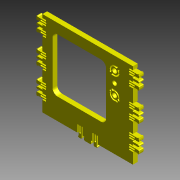
# Autodesk Inventor part: sideA
Saved by Autodesk Inventor 2012 (Build 160160000, 160)
## iProperties
Created: 2011-10-14
Part Number: sideA
Document SubType Name: Modeling
Designer: cramera
Density: 0.952 g/cm^3
Material: High Density Polyethylene
Mass: 352.422 g
Surface Area: 1032.73 cm^2
Volume: 370.191 cm^3
Autodesk Inventor part; units mm, degrees
ref_plane "YZ Plane" through (0, 0, 0) normal (1, 0, 0) x (0, 1, 0)
ref_plane "XZ Plane" through (0, 0, 0) normal (0, 1, 0) x (-1, 0, 0)
ref_plane "XY Plane" through (0, 0, 0) normal (0, 0, 1) x (1, 0, 0)
derived "skeleton.ipt"
sketch "POCKET_1-16" plane through (0, 0, 0) normal (0, 0, 1) x (1, 0, 0)
  circle A0 centre (239.1243, 767.2962) radius 7.3977
  constraints: 1 centre point
sketch "STOCK_12MM" plane through (0, 0, 0) normal (0, 0, 1) x (1, 0, 0)
  line L0 (457.2, 914.4) -> (457.2, 0)
  line L1 (0, 0) -> (457.2, 0)
  line L2 (457.2, 0) -> (457.2, 914.4)
  line L3 (457.2, 914.4) -> (0, 914.4)
  line L4 (0, 914.4) -> (0, 0)
  constraints: 10 end point
sketch "THROUGH-CUT" plane through (0, 0, 0) normal (0, 0, 1) x (1, 0, 0)
  line L0 (94.6618, 802.2212) -> (204.8343, 802.2212)
  arc A0 (217.5343, 789.5212) -> (204.8343, 802.2212) centre (204.8343, 789.5212) ccw
  line L1 (217.5343, 789.5212) -> (217.5343, 678.3962)
  arc A1 (204.8343, 665.6962) -> (217.5343, 678.3962) centre (204.8343, 678.3962) ccw
  line L2 (204.8343, 665.6962) -> (94.6618, 665.6962)
  arc A2 (81.9618, 678.3962) -> (94.6618, 665.6962) centre (94.6618, 678.3962) ccw
  line L3 (81.9618, 678.3962) -> (81.9618, 789.5212)
  arc A3 (94.6618, 802.2212) -> (81.9618, 789.5212) centre (94.6618, 789.5212) ccw
  circle A4 centre (239.1243, 794.2837) radius 5.925
  circle A5 centre (239.1243, 740.3087) radius 5.925
  circle A6 centre (239.1243, 767.2962) radius 5.5563
  arc A7 (51.3833, 713.1307) -> (52.9708, 711.5432) centre (52.9708, 713.1307) ccw
  line L4 (52.9708, 711.5432) -> (64.4993, 711.5432)
  arc A8 (64.4993, 711.5432) -> (66.0868, 713.1307) centre (64.4993, 713.1307) ccw
  line L5 (66.0868, 713.1307) -> (66.0868, 713.2577)
  arc A9 (66.0868, 713.2577) -> (64.4993, 714.8452) centre (64.4993, 713.2577) ccw
  line L6 (64.4993, 714.8452) -> (52.9708, 714.8452)
  arc A10 (52.9708, 714.8452) -> (51.3833, 713.2577) centre (52.9708, 713.2577) ccw
  line L7 (51.3833, 713.2577) -> (51.3833, 713.1307)
  arc A11 (277.2243, 673.8242) -> (275.6368, 672.2367) centre (277.2243, 672.2367) ccw
  line L8 (275.6368, 672.2367) -> (275.6368, 672.1097)
  arc A12 (275.6368, 672.1097) -> (277.2243, 670.5222) centre (277.2243, 672.1097) ccw
  line L9 (277.2243, 670.5222) -> (288.7527, 670.5222)
  arc A13 (288.7527, 670.5222) -> (290.3402, 672.1097) centre (288.7527, 672.1097) ccw
  line L10 (290.3402, 672.1097) -> (290.3402, 672.2367)
  arc A14 (290.3402, 672.2367) -> (288.7527, 673.8242) centre (288.7527, 672.2367) ccw
  line L11 (288.7527, 673.8242) -> (277.2243, 673.8242)
  arc A15 (277.2243, 740.4992) -> (275.6368, 738.9117) centre (277.2243, 738.9117) ccw
  line L12 (275.6368, 738.9117) -> (275.6368, 738.7847)
  arc A16 (275.6368, 738.7847) -> (277.2243, 737.1972) centre (277.2243, 738.7847) ccw
  line L13 (277.2243, 737.1972) -> (288.7527, 737.1972)
  arc A17 (288.7527, 737.1972) -> (290.3402, 738.7847) centre (288.7527, 738.7847) ccw
  line L14 (290.3402, 738.7847) -> (290.3402, 738.9117)
  arc A18 (290.3402, 738.9117) -> (288.7527, 740.4992) centre (288.7527, 738.9117) ccw
  line L15 (288.7527, 740.4992) -> (277.2243, 740.4992)
  line L16 (148.0018, 609.2685) -> (148.0018, 606.6412)
  line L17 (148.0018, 606.6412) -> (146.4778, 605.3712)
  line L18 (146.4778, 605.3712) -> (146.4778, 603.6533)
  line L19 (146.4778, 603.6533) -> (150.0773, 602.8312)
  line L20 (150.0773, 602.8312) -> (153.7803, 602.8312)
  arc A19 (153.7803, 602.8312) -> (155.3678, 604.4187) centre (153.7803, 604.4187) ccw
  line L21 (155.3678, 604.4187) -> (155.3678, 629.1837)
  arc A20 (156.9553, 630.7712) -> (155.3678, 629.1837) centre (156.9553, 629.1837) ccw
  line L22 (156.9553, 630.7712) -> (157.0823, 630.7712)
  arc A21 (158.6698, 629.1837) -> (157.0823, 630.7712) centre (157.0823, 629.1837) ccw
  line L23 (158.6698, 629.1837) -> (158.6698, 611.7212)
  line L24 (158.6698, 611.7212) -> (159.7267, 611.7212)
  arc A22 (161.9718, 609.4762) -> (159.7267, 611.7212) centre (160.8493, 610.5987) ccw
  line L25 (161.9718, 609.4762) -> (161.9718, 604.4187)
  line L26 (161.9718, 604.4187) -> (163.5593, 602.8312)
  line L27 (163.5593, 602.8312) -> (178.1643, 602.8312)
  line L28 (178.1643, 602.8312) -> (179.7518, 604.4187)
  line L29 (179.7518, 604.4187) -> (179.7518, 609.4762)
  arc A23 (181.9968, 611.7212) -> (179.7518, 609.4762) centre (180.8743, 610.5987) ccw
  line L30 (181.9968, 611.7212) -> (183.0538, 611.7212)
  line L31 (183.0538, 611.7212) -> (183.0538, 629.1837)
  arc A24 (184.6413, 630.7712) -> (183.0538, 629.1837) centre (184.6413, 629.1837) ccw
  line L32 (184.6413, 630.7712) -> (184.7604, 630.7712)
  arc A25 (186.3479, 629.1837) -> (184.7604, 630.7712) centre (184.7604, 629.1837) ccw
  line L33 (186.3479, 629.1837) -> (186.3558, 604.4187)
  arc A26 (186.3558, 604.4187) -> (187.9411, 602.8312) centre (187.9433, 604.4187) ccw
  line L34 (187.9411, 602.8312) -> (191.6462, 602.8312)
  line L35 (191.6462, 602.8312) -> (195.2458, 603.6533)
  line L36 (195.2458, 603.6533) -> (195.2458, 605.3712)
  line L37 (195.2458, 605.3712) -> (193.7218, 606.6412)
  line L38 (193.7218, 606.6412) -> (193.7218, 609.2685)
  line L39 (193.7218, 609.2685) -> (193.7218, 629.1837)
  arc A27 (195.3093, 630.7712) -> (193.7218, 629.1837) centre (195.3093, 629.1837) ccw
  line L40 (195.3093, 630.7712) -> (195.4363, 630.7712)
  arc A28 (197.0238, 629.1837) -> (195.4363, 630.7712) centre (195.4363, 629.1837) ccw
  line L41 (197.0238, 629.1837) -> (197.0238, 611.7212)
  line L42 (197.0238, 611.7212) -> (285.5428, 611.7212)
  line L43 (285.5428, 611.7212) -> (285.5428, 639.5342)
  line L44 (285.5428, 639.5342) -> (277.6053, 639.5342)
  arc A29 (276.0178, 641.1217) -> (277.6053, 639.5342) centre (277.6053, 641.1217) ccw
  line L45 (276.0178, 641.1217) -> (276.0178, 641.2487)
  arc A30 (277.6053, 642.8362) -> (276.0178, 641.2487) centre (277.6053, 641.2487) ccw
  line L46 (277.6053, 642.8362) -> (294.3455, 642.8362)
  line L47 (294.3455, 642.8362) -> (296.9728, 642.8362)
  line L48 (296.9728, 642.8362) -> (298.2428, 641.3122)
  line L49 (298.2428, 641.3122) -> (299.9607, 641.3122)
  line L50 (299.9607, 641.3122) -> (300.7828, 644.9118)
  line L51 (300.7828, 644.9118) -> (300.7828, 648.6169)
  arc A31 (300.7828, 648.6169) -> (299.1953, 650.2022) centre (299.1953, 648.6147) ccw
  line L52 (299.1953, 650.2022) -> (277.6053, 650.2022)
  arc A32 (276.0178, 651.7897) -> (277.6053, 650.2022) centre (277.6053, 651.7897) ccw
  line L53 (276.0178, 651.7897) -> (276.0178, 651.9167)
  arc A33 (277.6053, 653.5042) -> (276.0178, 651.9167) centre (277.6053, 651.9167) ccw
  line L54 (277.6053, 653.5042) -> (285.5428, 653.5042)
  line L55 (285.5428, 653.5042) -> (285.5428, 654.5612)
  arc A34 (285.5428, 656.8062) -> (285.5428, 654.5612) centre (286.6653, 655.6837) ccw
  arc A35 (287.7878, 656.8062) -> (285.5428, 656.8062) centre (286.6653, 655.6837) ccw
  line L56 (287.7878, 656.8062) -> (299.1953, 656.8062)
  line L57 (299.1953, 656.8062) -> (300.7828, 658.3937)
  line L58 (300.7828, 658.3937) -> (300.7828, 660.2987)
  line L59 (300.7828, 660.2987) -> (299.1953, 661.8862)
  line L60 (299.1953, 661.8862) -> (287.7878, 661.8862)
  arc A36 (285.5428, 661.8862) -> (287.7878, 661.8862) centre (286.6653, 663.0088) ccw
  arc A37 (285.5428, 664.1313) -> (285.5428, 661.8862) centre (286.6653, 663.0088) ccw
  line L61 (285.5428, 664.1313) -> (285.5428, 665.1882)
  line L62 (285.5428, 665.1882) -> (277.6053, 665.1882)
  arc A38 (276.0178, 666.7757) -> (277.6053, 665.1882) centre (277.6053, 666.7757) ccw
  line L63 (276.0178, 666.7757) -> (276.0178, 666.9027)
  arc A39 (277.6053, 668.4902) -> (276.0178, 666.9027) centre (277.6053, 666.9027) ccw
  line L64 (277.6053, 668.4902) -> (299.1953, 668.4902)
  arc A40 (299.1953, 668.4902) -> (300.7828, 670.0777) centre (299.1953, 670.0777) ccw
  line L65 (300.7828, 670.0777) -> (300.7828, 673.7807)
  line L66 (300.7828, 673.7807) -> (299.9607, 677.3802)
  line L67 (299.9607, 677.3802) -> (298.2428, 677.3802)
  line L68 (298.2428, 677.3802) -> (296.9728, 675.8562)
  line L69 (296.9728, 675.8562) -> (294.3455, 675.8562)
  line L70 (294.3455, 675.8562) -> (277.6053, 675.8562)
  arc A41 (276.0178, 677.4437) -> (277.6053, 675.8562) centre (277.6053, 677.4437) ccw
  line L71 (276.0178, 677.4437) -> (276.0178, 677.5707)
  arc A42 (277.6053, 679.1582) -> (276.0178, 677.5707) centre (277.6053, 677.5707) ccw
  line L72 (277.6053, 679.1582) -> (285.5428, 679.1582)
  line L73 (285.5428, 679.1582) -> (285.5428, 706.2092)
  line L74 (285.5428, 706.2092) -> (277.6053, 706.2092)
  arc A43 (276.0178, 707.7967) -> (277.6053, 706.2092) centre (277.6053, 707.7967) ccw
  line L75 (276.0178, 707.7967) -> (276.0178, 707.9237)
  arc A44 (277.6053, 709.5112) -> (276.0178, 707.9237) centre (277.6053, 707.9237) ccw
  line L76 (277.6053, 709.5112) -> (294.3455, 709.5112)
  line L77 (294.3455, 709.5112) -> (296.9728, 709.5112)
  line L78 (296.9728, 709.5112) -> (298.2428, 707.9872)
  line L79 (298.2428, 707.9872) -> (299.9607, 707.9872)
  line L80 (299.9607, 707.9872) -> (300.7828, 711.5868)
  line L81 (300.7828, 711.5868) -> (300.7828, 715.2919)
  arc A45 (300.7828, 715.2919) -> (299.1953, 716.8772) centre (299.1953, 715.2897) ccw
  line L82 (299.1953, 716.8772) -> (277.6053, 716.8772)
  arc A46 (276.0178, 718.4647) -> (277.6053, 716.8772) centre (277.6053, 718.4647) ccw
  line L83 (276.0178, 718.4647) -> (276.0178, 718.5917)
  arc A47 (277.6053, 720.1792) -> (276.0178, 718.5917) centre (277.6053, 718.5917) ccw
  line L84 (277.6053, 720.1792) -> (285.5428, 720.1792)
  line L85 (285.5428, 720.1792) -> (285.5428, 721.2362)
  arc A48 (285.5428, 723.4812) -> (285.5428, 721.2362) centre (286.6653, 722.3587) ccw
  arc A49 (287.7878, 723.4812) -> (285.5428, 723.4812) centre (286.6653, 722.3587) ccw
  line L86 (287.7878, 723.4812) -> (299.1953, 723.4812)
  line L87 (299.1953, 723.4812) -> (300.7828, 725.0687)
  line L88 (300.7828, 725.0687) -> (300.7828, 726.9737)
  line L89 (300.7828, 726.9737) -> (299.1953, 728.5612)
  line L90 (299.1953, 728.5612) -> (287.7878, 728.5612)
  arc A50 (285.5428, 728.5612) -> (287.7878, 728.5612) centre (286.6653, 729.6838) ccw
  arc A51 (285.5428, 730.8063) -> (285.5428, 728.5612) centre (286.6653, 729.6838) ccw
  line L91 (285.5428, 730.8063) -> (285.5428, 731.8632)
  line L92 (285.5428, 731.8632) -> (277.6053, 731.8632)
  arc A52 (276.0178, 733.4507) -> (277.6053, 731.8632) centre (277.6053, 733.4507) ccw
  line L93 (276.0178, 733.4507) -> (276.0178, 733.5777)
  arc A53 (277.6053, 735.1652) -> (276.0178, 733.5777) centre (277.6053, 733.5777) ccw
  line L94 (277.6053, 735.1652) -> (299.1953, 735.1652)
  arc A54 (299.1953, 735.1652) -> (300.7828, 736.7527) centre (299.1953, 736.7527) ccw
  line L95 (300.7828, 736.7527) -> (300.7828, 740.4557)
  line L96 (300.7828, 740.4557) -> (299.9607, 744.0552)
  line L97 (299.9607, 744.0552) -> (298.2428, 744.0552)
  line L98 (298.2428, 744.0552) -> (296.9728, 742.5312)
  line L99 (296.9728, 742.5312) -> (294.3455, 742.5312)
  line L100 (294.3455, 742.5312) -> (277.6053, 742.5312)
  arc A55 (276.0178, 744.1187) -> (277.6053, 742.5312) centre (277.6053, 744.1187) ccw
  line L101 (276.0178, 744.1187) -> (276.0178, 744.2457)
  arc A56 (277.6053, 745.8332) -> (276.0178, 744.2457) centre (277.6053, 744.2457) ccw
  line L102 (277.6053, 745.8332) -> (285.5428, 745.8332)
  line L103 (285.5428, 745.8332) -> (285.5428, 779.2342)
  line L104 (285.5428, 779.2342) -> (277.6053, 779.2342)
  arc A57 (276.0178, 780.8217) -> (277.6053, 779.2342) centre (277.6053, 780.8217) ccw
  line L105 (276.0178, 780.8217) -> (276.0178, 780.9487)
  arc A58 (277.6053, 782.5362) -> (276.0178, 780.9487) centre (277.6053, 780.9487) ccw
  line L106 (277.6053, 782.5362) -> (294.3455, 782.5362)
  line L107 (294.3455, 782.5362) -> (296.9728, 782.5362)
  line L108 (296.9728, 782.5362) -> (298.2428, 781.0122)
  line L109 (298.2428, 781.0122) -> (299.9607, 781.0122)
  line L110 (299.9607, 781.0122) -> (300.7828, 784.6118)
  line L111 (300.7828, 784.6118) -> (300.7828, 788.3169)
  arc A59 (300.7828, 788.3169) -> (299.1953, 789.9022) centre (299.1953, 788.3147) ccw
  line L112 (299.1953, 789.9022) -> (277.6053, 789.9022)
  arc A60 (276.0178, 791.4897) -> (277.6053, 789.9022) centre (277.6053, 791.4897) ccw
  line L113 (276.0178, 791.4897) -> (276.0178, 791.6167)
  arc A61 (277.6053, 793.2042) -> (276.0178, 791.6167) centre (277.6053, 791.6167) ccw
  line L114 (277.6053, 793.2042) -> (285.5428, 793.2042)
  line L115 (285.5428, 793.2042) -> (285.5428, 794.2612)
  arc A62 (285.5428, 796.5062) -> (285.5428, 794.2612) centre (286.6653, 795.3837) ccw
  arc A63 (287.7878, 796.5062) -> (285.5428, 796.5062) centre (286.6653, 795.3837) ccw
  line L116 (287.7878, 796.5062) -> (299.1953, 796.5062)
  line L117 (299.1953, 796.5062) -> (300.7828, 798.0937)
  line L118 (300.7828, 798.0937) -> (300.7828, 799.9987)
  line L119 (300.7828, 799.9987) -> (299.1953, 801.5862)
  line L120 (299.1953, 801.5862) -> (287.7878, 801.5862)
  arc A64 (285.5428, 801.5862) -> (287.7878, 801.5862) centre (286.6653, 802.7088) ccw
  arc A65 (285.5428, 803.8313) -> (285.5428, 801.5862) centre (286.6653, 802.7088) ccw
  line L121 (285.5428, 803.8313) -> (285.5428, 804.8882)
  line L122 (285.5428, 804.8882) -> (277.6053, 804.8882)
  arc A66 (276.0178, 806.4757) -> (277.6053, 804.8882) centre (277.6053, 806.4757) ccw
  line L123 (276.0178, 806.4757) -> (276.0178, 806.6027)
  arc A67 (277.6053, 808.1902) -> (276.0178, 806.6027) centre (277.6053, 806.6027) ccw
  line L124 (277.6053, 808.1902) -> (299.1953, 808.1902)
  arc A68 (299.1953, 808.1902) -> (300.7828, 809.7777) centre (299.1953, 809.7777) ccw
  line L125 (300.7828, 809.7777) -> (300.7828, 813.4807)
  line L126 (300.7828, 813.4807) -> (299.9607, 817.0802)
  line L127 (299.9607, 817.0802) -> (298.2428, 817.0802)
  line L128 (298.2428, 817.0802) -> (296.9728, 815.5562)
  line L129 (296.9728, 815.5562) -> (294.3455, 815.5562)
  line L130 (294.3455, 815.5562) -> (277.6053, 815.5562)
  arc A69 (276.0178, 817.1437) -> (277.6053, 815.5562) centre (277.6053, 817.1437) ccw
  line L131 (276.0178, 817.1437) -> (276.0178, 817.2707)
  arc A70 (277.6053, 818.8582) -> (276.0178, 817.2707) centre (277.6053, 817.2707) ccw
  line L132 (277.6053, 818.8582) -> (285.5428, 818.8582)
  line L133 (285.5428, 818.8582) -> (285.5428, 827.6212)
  line L134 (285.5428, 827.6212) -> (56.1808, 827.6212)
  line L135 (56.1808, 827.6212) -> (56.1808, 818.8582)
  line L136 (56.1808, 818.8582) -> (65.7058, 818.8582)
  line L137 (65.7058, 818.8582) -> (65.7058, 815.5562)
  line L138 (65.7058, 815.5562) -> (47.3781, 815.5562)
  line L139 (47.3781, 815.5562) -> (44.7508, 815.5562)
  line L140 (44.7508, 815.5562) -> (43.4808, 817.0802)
  line L141 (43.4808, 817.0802) -> (41.7629, 817.0802)
  line L142 (41.7629, 817.0802) -> (40.9408, 813.4807)
  line L143 (40.9408, 813.4807) -> (40.9408, 809.7777)
  arc A71 (40.9408, 809.7777) -> (42.5283, 808.1902) centre (42.5283, 809.7777) ccw
  line L144 (42.5283, 808.1902) -> (64.1183, 808.1902)
  arc A72 (65.7058, 806.6027) -> (64.1183, 808.1902) centre (64.1183, 806.6027) ccw
  line L145 (65.7058, 806.6027) -> (65.7058, 806.4757)
  arc A73 (64.1183, 804.8882) -> (65.7058, 806.4757) centre (64.1183, 806.4757) ccw
  line L146 (64.1183, 804.8882) -> (56.1808, 804.8882)
  line L147 (56.1808, 804.8882) -> (56.1808, 803.8313)
  arc A74 (53.9357, 801.5862) -> (56.1808, 803.8313) centre (55.0583, 802.7088) ccw
  line L148 (53.9357, 801.5862) -> (42.5283, 801.5862)
  line L149 (42.5283, 801.5862) -> (40.9408, 799.9987)
  line L150 (40.9408, 799.9987) -> (40.9408, 798.0937)
  line L151 (40.9408, 798.0937) -> (42.5283, 796.5062)
  line L152 (42.5283, 796.5062) -> (53.9357, 796.5062)
  arc A75 (56.1808, 794.2612) -> (53.9357, 796.5062) centre (55.0583, 795.3837) ccw
  line L153 (56.1808, 794.2612) -> (56.1808, 793.2042)
  line L154 (56.1808, 793.2042) -> (64.1183, 793.2042)
  arc A76 (65.7058, 791.6167) -> (64.1183, 793.2042) centre (64.1183, 791.6167) ccw
  line L155 (65.7058, 791.6167) -> (65.7058, 791.4897)
  arc A77 (64.1183, 789.9022) -> (65.7058, 791.4897) centre (64.1183, 791.4897) ccw
  line L156 (64.1183, 789.9022) -> (42.5283, 789.9022)
  arc A78 (42.5283, 789.9022) -> (40.9408, 788.3169) centre (42.5283, 788.3147) ccw
  line L157 (40.9408, 788.3169) -> (40.9408, 784.6118)
  line L158 (40.9408, 784.6118) -> (41.7629, 781.0122)
  line L159 (41.7629, 781.0122) -> (43.4808, 781.0122)
  line L160 (43.4808, 781.0122) -> (44.7508, 782.5362)
  line L161 (44.7508, 782.5362) -> (47.3781, 782.5362)
  line L162 (47.3781, 782.5362) -> (64.1183, 782.5362)
  arc A79 (65.7058, 780.9487) -> (64.1183, 782.5362) centre (64.1183, 780.9487) ccw
  line L163 (65.7058, 780.9487) -> (65.7058, 780.8217)
  arc A80 (64.1183, 779.2342) -> (65.7058, 780.8217) centre (64.1183, 780.8217) ccw
  line L164 (64.1183, 779.2342) -> (56.1808, 779.2342)
  line L165 (56.1808, 779.2342) -> (56.1808, 745.8332)
  line L166 (56.1808, 745.8332) -> (64.1183, 745.8332)
  arc A81 (65.7058, 744.2457) -> (64.1183, 745.8332) centre (64.1183, 744.2457) ccw
  line L167 (65.7058, 744.2457) -> (65.7058, 744.1187)
  arc A82 (64.1183, 742.5312) -> (65.7058, 744.1187) centre (64.1183, 744.1187) ccw
  line L168 (64.1183, 742.5312) -> (47.3781, 742.5312)
  line L169 (47.3781, 742.5312) -> (44.7508, 742.5312)
  line L170 (44.7508, 742.5312) -> (43.4808, 744.0552)
  line L171 (43.4808, 744.0552) -> (41.7629, 744.0552)
  line L172 (41.7629, 744.0552) -> (40.9408, 740.4557)
  line L173 (40.9408, 740.4557) -> (40.9408, 736.7527)
  arc A83 (40.9408, 736.7527) -> (42.5283, 735.1652) centre (42.5283, 736.7527) ccw
  line L174 (42.5283, 735.1652) -> (64.1183, 735.1652)
  arc A84 (65.7058, 733.5777) -> (64.1183, 735.1652) centre (64.1183, 733.5777) ccw
  line L175 (65.7058, 733.5777) -> (65.7058, 733.4507)
  arc A85 (64.1183, 731.8632) -> (65.7058, 733.4507) centre (64.1183, 733.4507) ccw
  line L176 (64.1183, 731.8632) -> (56.1808, 731.8632)
  line L177 (56.1808, 731.8632) -> (56.1808, 730.8063)
  arc A86 (53.9357, 728.5612) -> (56.1808, 730.8063) centre (55.0583, 729.6838) ccw
  line L178 (53.9357, 728.5612) -> (42.5283, 728.5612)
  line L179 (42.5283, 728.5612) -> (40.9408, 726.9737)
  line L180 (40.9408, 726.9737) -> (40.9408, 725.0687)
  line L181 (40.9408, 725.0687) -> (42.5283, 723.4812)
  line L182 (42.5283, 723.4812) -> (53.9357, 723.4812)
  arc A87 (56.1808, 721.2362) -> (53.9357, 723.4812) centre (55.0583, 722.3587) ccw
  line L183 (56.1808, 721.2362) -> (56.1808, 720.1792)
  line L184 (56.1808, 720.1792) -> (64.1183, 720.1792)
  arc A88 (65.7058, 718.5917) -> (64.1183, 720.1792) centre (64.1183, 718.5917) ccw
  line L185 (65.7058, 718.5917) -> (65.7058, 718.4647)
  arc A89 (64.1183, 716.8772) -> (65.7058, 718.4647) centre (64.1183, 718.4647) ccw
  line L186 (64.1183, 716.8772) -> (42.5283, 716.8772)
  arc A90 (42.5283, 716.8772) -> (40.9408, 715.2919) centre (42.5283, 715.2897) ccw
  line L187 (40.9408, 715.2919) -> (40.9408, 711.5868)
  line L188 (40.9408, 711.5868) -> (41.7629, 707.9872)
  line L189 (41.7629, 707.9872) -> (43.4808, 707.9872)
  line L190 (43.4808, 707.9872) -> (44.7508, 709.5112)
  line L191 (44.7508, 709.5112) -> (47.3781, 709.5112)
  line L192 (47.3781, 709.5112) -> (64.1183, 709.5112)
  arc A91 (65.7058, 707.9237) -> (64.1183, 709.5112) centre (64.1183, 707.9237) ccw
  line L193 (65.7058, 707.9237) -> (65.7058, 707.7967)
  arc A92 (64.1183, 706.2092) -> (65.7058, 707.7967) centre (64.1183, 707.7967) ccw
  line L194 (64.1183, 706.2092) -> (56.1808, 706.2092)
  line L195 (56.1808, 706.2092) -> (56.1808, 679.1582)
  line L196 (56.1808, 679.1582) -> (64.1183, 679.1582)
  arc A93 (65.7058, 677.5707) -> (64.1183, 679.1582) centre (64.1183, 677.5707) ccw
  line L197 (65.7058, 677.5707) -> (65.7058, 677.4437)
  arc A94 (64.1183, 675.8562) -> (65.7058, 677.4437) centre (64.1183, 677.4437) ccw
  line L198 (64.1183, 675.8562) -> (47.3781, 675.8562)
  line L199 (47.3781, 675.8562) -> (44.7508, 675.8562)
  line L200 (44.7508, 675.8562) -> (43.4808, 677.3802)
  line L201 (43.4808, 677.3802) -> (41.7629, 677.3802)
  line L202 (41.7629, 677.3802) -> (40.9408, 673.7807)
  line L203 (40.9408, 673.7807) -> (40.9408, 670.0777)
  arc A95 (40.9408, 670.0777) -> (42.5283, 668.4902) centre (42.5283, 670.0777) ccw
  line L204 (42.5283, 668.4902) -> (64.1183, 668.4902)
  arc A96 (65.7058, 666.9027) -> (64.1183, 668.4902) centre (64.1183, 666.9027) ccw
  line L205 (65.7058, 666.9027) -> (65.7058, 666.7757)
  arc A97 (64.1183, 665.1882) -> (65.7058, 666.7757) centre (64.1183, 666.7757) ccw
  line L206 (64.1183, 665.1882) -> (56.1808, 665.1882)
  line L207 (56.1808, 665.1882) -> (56.1808, 664.1313)
  arc A98 (53.9357, 661.8862) -> (56.1808, 664.1313) centre (55.0583, 663.0088) ccw
  line L208 (53.9357, 661.8862) -> (42.5283, 661.8862)
  line L209 (42.5283, 661.8862) -> (40.9408, 660.2987)
  line L210 (40.9408, 660.2987) -> (40.9408, 658.3937)
  line L211 (40.9408, 658.3937) -> (42.5283, 656.8062)
  line L212 (42.5283, 656.8062) -> (53.9357, 656.8062)
  arc A99 (56.1808, 654.5612) -> (53.9357, 656.8062) centre (55.0583, 655.6837) ccw
  line L213 (56.1808, 654.5612) -> (56.1808, 653.5042)
  line L214 (56.1808, 653.5042) -> (64.1087, 653.5042)
  arc A100 (65.6962, 651.9167) -> (64.1087, 653.5042) centre (64.1087, 651.9167) ccw
  line L215 (65.6962, 651.9167) -> (65.7058, 651.7897)
  arc A101 (64.1183, 650.2022) -> (65.7058, 651.7897) centre (64.1183, 651.7897) ccw
  line L216 (64.1183, 650.2022) -> (42.5283, 650.2022)
  arc A102 (42.5283, 650.2022) -> (40.9408, 648.6169) centre (42.5283, 648.6147) ccw
  line L217 (40.9408, 648.6169) -> (40.9408, 644.9118)
  line L218 (40.9408, 644.9118) -> (41.7629, 641.3122)
  line L219 (41.7629, 641.3122) -> (43.4808, 641.3122)
  line L220 (43.4808, 641.3122) -> (44.7508, 642.8362)
  line L221 (44.7508, 642.8362) -> (47.3781, 642.8362)
  line L222 (47.3781, 642.8362) -> (64.1183, 642.8362)
  arc A103 (65.7058, 641.2487) -> (64.1183, 642.8362) centre (64.1183, 641.2487) ccw
  line L223 (65.7058, 641.2487) -> (65.7058, 641.1217)
  arc A104 (64.1183, 639.5342) -> (65.7058, 641.1217) centre (64.1183, 641.1217) ccw
  line L224 (64.1183, 639.5342) -> (56.1808, 639.5342)
  line L225 (56.1808, 639.5342) -> (56.1808, 611.7212)
  line L226 (56.1808, 611.7212) -> (144.6998, 611.7212)
  line L227 (144.6998, 611.7212) -> (144.6998, 629.1837)
  arc A105 (146.2873, 630.7712) -> (144.6998, 629.1837) centre (146.2873, 629.1837) ccw
  line L228 (146.2873, 630.7712) -> (146.4143, 630.7712)
  arc A106 (148.0018, 629.1837) -> (146.4143, 630.7712) centre (146.4143, 629.1837) ccw
  line L229 (148.0018, 629.1837) -> (148.0018, 609.2685)
  arc A107 (277.2243, 648.1702) -> (275.6368, 646.5827) centre (277.2243, 646.5827) ccw
  line L230 (277.2243, 648.1702) -> (288.7527, 648.1702)
  arc A108 (290.3402, 646.5827) -> (288.7527, 648.1702) centre (288.7527, 646.5827) ccw
  line L231 (290.3402, 646.5827) -> (290.3402, 646.4557)
  arc A109 (288.7527, 644.8682) -> (290.3402, 646.4557) centre (288.7527, 646.4557) ccw
  line L232 (288.7527, 644.8682) -> (277.2243, 644.8682)
  arc A110 (275.6368, 646.4557) -> (277.2243, 644.8682) centre (277.2243, 646.4557) ccw
  line L233 (275.6368, 646.4557) -> (275.6368, 646.5827)
  arc A111 (52.9708, 673.8242) -> (51.3833, 672.2367) centre (52.9708, 672.2367) ccw
  line L234 (52.9708, 673.8242) -> (64.4993, 673.8242)
  arc A112 (66.0868, 672.2367) -> (64.4993, 673.8242) centre (64.4993, 672.2367) ccw
  line L235 (66.0868, 672.2367) -> (66.0868, 672.1097)
  arc A113 (64.4993, 670.5222) -> (66.0868, 672.1097) centre (64.4993, 672.1097) ccw
  line L236 (64.4993, 670.5222) -> (52.9708, 670.5222)
  arc A114 (51.3833, 672.1097) -> (52.9708, 670.5222) centre (52.9708, 672.1097) ccw
  line L237 (51.3833, 672.1097) -> (51.3833, 672.2367)
  arc A115 (227.7837, 744.5729) -> (243.3885, 728.9681) centre (239.1243, 740.3087) ccw
  line L238 (243.3885, 728.9681) -> (244.0601, 728.2965)
  arc A116 (244.0601, 728.2965) -> (246.3051, 728.2965) centre (245.1826, 729.419) ccw
  line L239 (246.3051, 728.2965) -> (246.377, 728.3683)
  arc A117 (246.377, 728.3683) -> (246.377, 730.6134) centre (245.2545, 729.4909) ccw
  line L240 (246.377, 730.6134) -> (244.8933, 732.0971)
  arc A118 (244.8933, 732.0971) -> (243.0633, 732.3957) centre (243.7707, 730.9746) ccw
  arc A119 (231.2113, 744.2478) -> (243.0633, 732.3957) centre (239.1243, 740.3087) ccw
  arc A120 (231.2113, 744.2478) -> (230.9127, 746.0777) centre (229.7901, 744.9552) ccw
  line L241 (230.9127, 746.0777) -> (229.429, 747.5614)
  arc A121 (229.429, 747.5614) -> (227.1839, 747.5614) centre (228.3064, 746.4389) ccw
  line L242 (227.1839, 747.5614) -> (227.112, 747.4896)
  arc A122 (227.112, 747.4896) -> (227.112, 745.2445) centre (228.2346, 746.3671) ccw
  line L243 (227.112, 745.2445) -> (227.7837, 744.5729)
  arc A123 (52.9708, 787.8702) -> (51.3833, 786.2827) centre (52.9708, 786.2827) ccw
  line L244 (51.3833, 786.2827) -> (51.3833, 786.1557)
  arc A124 (51.3833, 786.1557) -> (52.9708, 784.5682) centre (52.9708, 786.1557) ccw
  line L245 (52.9708, 784.5682) -> (64.4993, 784.5682)
  arc A125 (64.4993, 784.5682) -> (66.0868, 786.1557) centre (64.4993, 786.1557) ccw
  line L246 (66.0868, 786.1557) -> (66.0868, 786.2827)
  arc A126 (66.0868, 786.2827) -> (64.4993, 787.8702) centre (64.4993, 786.2827) ccw
  line L247 (64.4993, 787.8702) -> (52.9708, 787.8702)
  arc A127 (247.0373, 736.3697) -> (247.3359, 734.5397) centre (248.4584, 735.6623) ccw
  line L248 (247.3359, 734.5397) -> (248.8196, 733.056)
  arc A128 (248.8196, 733.056) -> (251.0647, 733.056) centre (249.9421, 734.1786) ccw
  line L249 (251.0647, 733.056) -> (251.1365, 733.1279)
  arc A129 (251.1365, 733.1279) -> (251.1365, 735.3729) centre (250.014, 734.2504) ccw
  line L250 (251.1365, 735.3729) -> (250.4649, 736.0446)
  arc A130 (250.4649, 736.0446) -> (234.8601, 751.6494) centre (239.1243, 740.3087) ccw
  line L251 (234.8601, 751.6494) -> (234.1885, 752.321)
  arc A131 (234.1885, 752.321) -> (231.9434, 752.321) centre (233.066, 751.1984) ccw
  line L252 (231.9434, 752.321) -> (231.8716, 752.2491)
  arc A132 (231.8716, 752.2491) -> (231.8716, 750.0041) centre (232.9941, 751.1266) ccw
  line L253 (231.8716, 750.0041) -> (233.3553, 748.5204)
  arc A133 (233.3553, 748.5204) -> (235.1853, 748.2217) centre (234.4778, 749.6429) ccw
  arc A134 (247.0373, 736.3697) -> (235.1853, 748.2217) centre (239.1243, 740.3087) ccw
  arc A135 (277.2243, 787.8702) -> (275.6368, 786.2827) centre (277.2243, 786.2827) ccw
  line L254 (277.2243, 787.8702) -> (288.7527, 787.8702)
  arc A136 (290.3402, 786.2827) -> (288.7527, 787.8702) centre (288.7527, 786.2827) ccw
  line L255 (290.3402, 786.2827) -> (290.3402, 786.1557)
  arc A137 (288.7527, 784.5682) -> (290.3402, 786.1557) centre (288.7527, 786.1557) ccw
  line L256 (288.7527, 784.5682) -> (277.2243, 784.5682)
  arc A138 (275.6368, 786.1557) -> (277.2243, 784.5682) centre (277.2243, 786.1557) ccw
  line L257 (275.6368, 786.1557) -> (275.6368, 786.2827)
  arc A139 (227.112, 789.3479) -> (227.112, 787.1029) centre (228.2346, 788.2254) ccw
  line L258 (227.112, 789.3479) -> (227.7837, 790.0196)
  arc A140 (243.3885, 805.6244) -> (227.7837, 790.0196) centre (239.1243, 794.2837) ccw
  line L259 (243.3885, 805.6244) -> (244.0601, 806.296)
  arc A141 (246.3051, 806.296) -> (244.0601, 806.296) centre (245.1826, 805.1734) ccw
  line L260 (246.3051, 806.296) -> (246.377, 806.2241)
  arc A142 (246.377, 803.9791) -> (246.377, 806.2241) centre (245.2545, 805.1016) ccw
  line L261 (246.377, 803.9791) -> (244.8933, 802.4954)
  arc A143 (243.0633, 802.1967) -> (244.8933, 802.4954) centre (243.7707, 803.6179) ccw
  arc A144 (243.0633, 802.1967) -> (231.2113, 790.3447) centre (239.1243, 794.2837) ccw
  arc A145 (230.9127, 788.5147) -> (231.2113, 790.3447) centre (229.7901, 789.6373) ccw
  line L262 (230.9127, 788.5147) -> (229.429, 787.031)
  arc A146 (227.1839, 787.031) -> (229.429, 787.031) centre (228.3064, 788.1536) ccw
  line L263 (227.1839, 787.031) -> (227.112, 787.1029)
  arc A147 (288.7527, 711.5432) -> (290.3402, 713.1307) centre (288.7527, 713.1307) ccw
  line L264 (288.7527, 711.5432) -> (277.2243, 711.5432)
  arc A148 (275.6368, 713.1307) -> (277.2243, 711.5432) centre (277.2243, 713.1307) ccw
  line L265 (275.6368, 713.1307) -> (275.6368, 713.2577)
  arc A149 (277.2243, 714.8452) -> (275.6368, 713.2577) centre (277.2243, 713.2577) ccw
  line L266 (277.2243, 714.8452) -> (288.7527, 714.8452)
  arc A150 (290.3402, 713.2577) -> (288.7527, 714.8452) centre (288.7527, 713.2577) ccw
  line L267 (290.3402, 713.2577) -> (290.3402, 713.1307)
  arc A151 (52.9708, 813.5242) -> (51.3833, 811.9367) centre (52.9708, 811.9367) ccw
  line L268 (52.9708, 813.5242) -> (64.4993, 813.5242)
  arc A152 (66.0868, 811.9367) -> (64.4993, 813.5242) centre (64.4993, 811.9367) ccw
  line L269 (66.0868, 811.9367) -> (66.0868, 811.8097)
  arc A153 (64.4993, 810.2222) -> (66.0868, 811.8097) centre (64.4993, 811.8097) ccw
  line L270 (64.4993, 810.2222) -> (52.9708, 810.2222)
  arc A154 (51.3833, 811.8097) -> (52.9708, 810.2222) centre (52.9708, 811.8097) ccw
  line L271 (51.3833, 811.8097) -> (51.3833, 811.9367)
  arc A155 (277.2243, 813.5242) -> (275.6368, 811.9367) centre (277.2243, 811.9367) ccw
  line L272 (275.6368, 811.9367) -> (275.6368, 811.8097)
  arc A156 (275.6368, 811.8097) -> (277.2243, 810.2222) centre (277.2243, 811.8097) ccw
  line L273 (277.2243, 810.2222) -> (288.7527, 810.2222)
  arc A157 (288.7527, 810.2222) -> (290.3402, 811.8097) centre (288.7527, 811.8097) ccw
  line L274 (290.3402, 811.8097) -> (290.3402, 811.9367)
  arc A158 (290.3402, 811.9367) -> (288.7527, 813.5242) centre (288.7527, 811.9367) ccw
  line L275 (288.7527, 813.5242) -> (277.2243, 813.5242)
  arc A159 (51.3833, 738.7847) -> (52.9708, 737.1972) centre (52.9708, 738.7847) ccw
  line L276 (51.3833, 738.7847) -> (51.3833, 738.9117)
  arc A160 (52.9708, 740.4992) -> (51.3833, 738.9117) centre (52.9708, 738.9117) ccw
  line L277 (52.9708, 740.4992) -> (64.4993, 740.4992)
  arc A161 (66.0868, 738.9117) -> (64.4993, 740.4992) centre (64.4993, 738.9117) ccw
  line L278 (66.0868, 738.9117) -> (66.0868, 738.7847)
  arc A162 (64.4993, 737.1972) -> (66.0868, 738.7847) centre (64.4993, 738.7847) ccw
  line L279 (64.4993, 737.1972) -> (52.9708, 737.1972)
  arc A163 (52.9708, 648.1702) -> (51.3833, 646.5827) centre (52.9708, 646.5827) ccw
  line L280 (51.3833, 646.5827) -> (51.3833, 646.4557)
  arc A164 (51.3833, 646.4557) -> (52.9708, 644.8682) centre (52.9708, 646.4557) ccw
  line L281 (52.9708, 644.8682) -> (64.4993, 644.8682)
  arc A165 (64.4993, 644.8682) -> (66.0868, 646.4557) centre (64.4993, 646.4557) ccw
  line L282 (66.0868, 646.4557) -> (66.0868, 646.5827)
  arc A166 (66.0868, 646.5827) -> (64.4993, 648.1702) centre (64.4993, 646.5827) ccw
  line L283 (64.4993, 648.1702) -> (52.9708, 648.1702)
  arc A167 (188.3878, 614.4803) -> (189.9753, 612.8928) centre (189.9753, 614.4803) ccw
  line L284 (189.9753, 612.8928) -> (190.1023, 612.8928)
  arc A168 (190.1023, 612.8928) -> (191.6898, 614.4803) centre (190.1023, 614.4803) ccw
  line L285 (191.6898, 614.4803) -> (191.6898, 629.1837)
  arc A169 (191.6898, 629.1837) -> (190.1023, 630.7712) centre (190.1023, 629.1837) ccw
  line L286 (190.1023, 630.7712) -> (189.9753, 630.7712)
  arc A170 (189.9753, 630.7712) -> (188.3878, 629.1837) centre (189.9753, 629.1837) ccw
  line L287 (188.3878, 629.1837) -> (188.3878, 614.4803)
  arc A171 (150.0338, 614.4803) -> (151.6213, 612.8928) centre (151.6213, 614.4803) ccw
  line L288 (150.0338, 614.4803) -> (150.0338, 629.1837)
  arc A172 (151.6213, 630.7712) -> (150.0338, 629.1837) centre (151.6213, 629.1837) ccw
  line L289 (151.6213, 630.7712) -> (151.7483, 630.7712)
  arc A173 (153.3358, 629.1837) -> (151.7483, 630.7712) centre (151.7483, 629.1837) ccw
  line L290 (153.3358, 629.1837) -> (153.3358, 614.4803)
  arc A174 (151.7483, 612.8928) -> (153.3358, 614.4803) centre (151.7483, 614.4803) ccw
  line L291 (151.7483, 612.8928) -> (151.6213, 612.8928)
  arc A175 (234.8601, 782.9431) -> (250.4649, 798.5479) centre (239.1243, 794.2837) ccw
  line L292 (234.8601, 782.9431) -> (234.1885, 782.2715)
  arc A176 (231.9434, 782.2715) -> (234.1885, 782.2715) centre (233.066, 783.394) ccw
  line L293 (231.9434, 782.2715) -> (231.8716, 782.3433)
  arc A177 (231.8716, 784.5884) -> (231.8716, 782.3433) centre (232.9941, 783.4659) ccw
  line L294 (231.8716, 784.5884) -> (233.3553, 786.0721)
  arc A178 (235.1853, 786.3707) -> (233.3553, 786.0721) centre (234.4778, 784.9496) ccw
  arc A179 (235.1853, 786.3707) -> (247.0373, 798.2228) centre (239.1243, 794.2837) ccw
  arc A180 (247.3359, 800.0527) -> (247.0373, 798.2228) centre (248.4584, 798.9302) ccw
  line L295 (247.3359, 800.0527) -> (248.8196, 801.5364)
  arc A181 (251.0647, 801.5364) -> (248.8196, 801.5364) centre (249.9421, 800.4139) ccw
  line L296 (251.0647, 801.5364) -> (251.1365, 801.4646)
  arc A182 (251.1365, 799.2195) -> (251.1365, 801.4646) centre (250.014, 800.3421) ccw
  line L297 (251.1365, 799.2195) -> (250.4649, 798.5479)
  dimension "d5" = 11.85
  dimension "d6" = 11.85
  constraints: 596 end point, 360 point on circle, 183 centre point
  measures "d5" diameter of A4
  measures "d6" diameter of A5
extrude "Extrusion1" add sketch "THROUGH-CUT" along normal blind 12
extrude "Extrusion2" cut sketch "POCKET_1-16" along normal blind 1.5875
equation "\"d6\" = d5"
equation "\"d1\" = StockThickness"
equation "\"StockThickness\" = 12"
body "Solid1"
